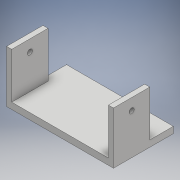
# Autodesk Inventor part: Ard for BR
Saved by Autodesk Inventor 2018.1 (Build 221171000, 171)
## iProperties
Created: 2019-02-17
Part Number: Ard for BR
Material: Типовые
Document SubType Name: Modeling
Designer: kostya
Density: 1 g/cm^3
Appearance: По умолчанию
Author: kostya
Autodesk Inventor part; units mm, degrees
ref_plane "YZ Plane" through (0, 0, 0) normal (1, 0, 0) x (0, 1, 0)
ref_plane "XZ Plane" through (0, 0, 0) normal (0, 1, 0) x (-1, 0, 0)
ref_plane "XY Plane" through (0, 0, 0) normal (0, 0, 1) x (1, 0, 0)
sketch "Эскиз1" plane through (0, 0, 0) normal (0, 0, 1) x (1, 0, 0)
  line L0 (-38, 52.38) -> (38, 52.38) construction
  line L1 (38, 52.38) -> (38, -52.38) construction
  line L2 (38, -52.38) -> (-38, -52.38) construction
  line L3 (-38, -52.38) -> (-38, 52.38) construction
  line L4 (-26.6205, -33.05) -> (26.6205, -33.05) construction
  line L5 (26.6205, -33.05) -> (26.6205, 33.05) construction
  line L6 (26.6205, 33.05) -> (-26.6205, 33.05) construction
  line L7 (-26.6205, 33.05) -> (-26.6205, -33.05) construction
  line L8 (0, 33.05) -> (0, 38.05) construction
  line L9 (0, -33.05) -> (0, -38.05) construction
  line L10 (-38, 38.05) -> (38, 38.05)
  line L11 (38, 38.05) -> (38, -38.05)
  line L12 (38, -38.05) -> (-38, -38.05)
  line L13 (-38, -38.05) -> (-38, 38.05)
  dimension "d0" = 76
  dimension "d1" = 104.76
  dimension "d2" = 53.241
  dimension "d3" = 66.1
  dimension "d4" = 5
  dimension "d5" = 5
  constraints: 28 end point, 6 parallel, 3 horizontal, 3 perpendicular, 2 midpoint, 2 point on line, 2 vertical
  measures "d0" distance of L1.end L2.end
  measures "d1" distance of L0.end L1.end
  measures "d2" distance of L6.end L5.end
  measures "d3" distance of L5.end L4.end
  measures "d4" distance of L8.start L8.end
  measures "d5" distance of L9.start L9.end
extrude "Выдавливание1" add sketch "Эскиз1" along normal blind 5
sketch "Эскиз2" plane through (0, 0, 5) normal (0, 0, 1) x (1, 0, 0)
  line L0 (38, 38.05) -> (38, -38.05) projected
  line L1 (-38, -38.05) -> (-38, 38.05) projected
  line L2 (-38, 38.05) -> (-38, -38.05) projected
  line L3 (-38, -38.05) -> (-42, -38.05)
  line L4 (38, 38.05) -> (42, 38.05)
  line L5 (42, -38.05) -> (42, 38.05)
  line L6 (-42, 38.05) -> (-42, -38.05)
  line L7 (-38, -38.05) -> (-38, 38.05)
  line L8 (38, 38.05) -> (-38, 38.05) projected
  line L9 (38, 38.05) -> (38, -38.05)
  line L10 (42, 38.05) -> (38, 38.05)
  line L11 (-38, 38.05) -> (-42, 38.05)
  line L12 (-42, -38.05) -> (-38, -38.05)
  line L13 (38, -38.05) -> (42, -38.05)
  point P0 (0, 0)
  dimension "d8" = 4
  dimension "d9" = 4
  constraints: 20 end point, 6 equal length, 4 horizontal, 4 perpendicular
  measures "d8" distance of L1.start L3.end
  measures "d9" distance of L0.start L4.end
extrude "Выдавливание2" add sketch "Эскиз2" along normal blind 24 and the other way blind 5
sketch "Эскиз3" plane through (0, 0, 29) normal (0, 0, 1) x (1, 0, 0)
  line L0 (38, 38.05) -> (38, -38.05) projected
  line L1 (38, -38.05) -> (42, -38.05) projected
  line L2 (42, -38.05) -> (42, 38.05) projected
  line L3 (42, 38.05) -> (38, 38.05) projected
  line L4 (42, 9.5) -> (38, 9.5)
  line L5 (38, 9.5) -> (38, -9.5)
  line L6 (38, -9.5) -> (42, -9.5)
  line L7 (42, -9.5) -> (42, 9.5)
  line L8 (42, 9.5) -> (38, -9.5) construction
  line L9 (38, 9.5) -> (42, -9.5) construction
  line L10 (0, 0) -> (0, -84) construction
  line L11 (-42, 9.5) -> (-38, 9.5)
  line L12 (-38, -9.5) -> (-42, -9.5)
  line L13 (-38, 9.5) -> (-38, -9.5) construction
  line L14 (-38, 38.05) -> (-38, -38.05) construction
  line L15 (-42, 9.5) -> (-42, -9.5) construction
  line L16 (-42, 38.05) -> (-42, -38.05) construction
  line L17 (-38, 9.5) -> (-38, -9.5)
  line L18 (-42, -9.5) -> (-42, 9.5)
  point P0 (40, 0)
  dimension "d14" = 4
  dimension "d15" = 19
  constraints: 26 end point, 4 symmetric about line, 3 collinear, 3 parallel, 2 midpoint, 1 horizontal, 1 perpendicular, 1 vertical
  measures "d14" distance of L6.end L5.end
  measures "d15" distance of L5.end L4.end
extrude "Выдавливание3" cut sketch "Эскиз3" against normal up to surface (24 mm away) contours L4 L2 L6 L0 | L11 L17 L12 L18
sketch "Эскиз4" plane through (-42, 38.05, 0) normal (0, 1, 0) x (1, 0, 0)
  line L0 (0, 0) -> (84, 0) projected
  line L1 (0, 0) -> (0, -29) projected
  line L2 (4, -29) -> (0, -29) projected
  line L3 (4, -29) -> (4, -5) projected
  line L4 (80, -5) -> (4, -5) projected
  line L5 (80, -29) -> (80, -5) projected
  line L6 (84, -29) -> (80, -29) projected
  line L7 (84, 0) -> (84, -29) projected
  point P0 (42, 0)
extrude "Выдавливание4" cut sketch "Эскиз4" against normal blind 29
sketch "Эскиз5" plane through (0, 0, 29) normal (0, 0, 1) x (1, 0, 0)
  line L0 (-38, -9.5) -> (-42, -9.5) projected
  line L1 (-42, -9.5) -> (-42, -38.05) projected
  line L2 (-42, -38.05) -> (-38, -38.05) projected
  line L3 (-38, -38.05) -> (-38, -9.5) projected
  line L4 (42, -9.5) -> (38, -9.5) projected
  line L5 (38, -9.5) -> (38, -38.05) projected
  line L6 (38, -38.05) -> (42, -38.05) projected
  line L7 (42, -38.05) -> (42, -9.5) projected
  point P0 (0, 0)
extrude "Выдавливание5" add sketch "Эскиз5" along normal blind 12
sketch "Эскиз6" plane through (42, -9.5, 5) normal (1, 0, 0) x (0, 0, -1)
  line L0 (5, 18.55) -> (0, 18.55) projected
  line L1 (0, 18.55) -> (0, 0) projected
  line L2 (0, 0) -> (-36, 0) projected
  line L3 (-36, -28.55) -> (-36, 0) projected
  line L4 (5, -28.55) -> (-36, -28.55) projected
  line L5 (5, 18.55) -> (5, -28.55) projected
  line L6 (-36, -28.55) -> (-36, 0) construction
  line L7 (-36, -14.275) -> (-27, -14.275) construction
  circle A0 centre (-27, -14.275) radius 2
  point P0 (5, 9.5)
  dimension "d22" = 9
  dimension "d23" = 4
  constraints: 2 end point, 1 centre point, 1 coincident, 1 horizontal, 1 midpoint
  measures "d22" distance of L7.start L7.end
  measures "d23" diameter of A0
extrude "Выдавливание6" cut sketch "Эскиз6" against normal up to surface (84 mm away) contours A0
